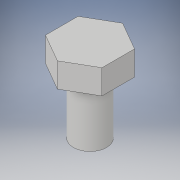
# Autodesk Inventor part: Crossbeam to LS Bolt
Saved by Autodesk Inventor 2017 (Build 210142000, 142)
## iProperties
Created: 2016-09-26
Part Number: Crossbeam to LS Bolt
Material: Generic
Document SubType Name: Modeling
Designer: Hanson
Density: 1 g/cm^3
Appearance: Default
Author: Hanson
Autodesk Inventor part; units mm, degrees
ref_plane "YZ Plane" through (0, 0, 0) normal (1, 0, 0) x (0, 1, 0)
ref_plane "XZ Plane" through (0, 0, 0) normal (0, 1, 0) x (-1, 0, 0)
ref_plane "XY Plane" through (0, 0, 0) normal (0, 0, 1) x (1, 0, 0)
sketch "Sketch1" plane through (0, 0, 0) normal (0, 1, 0) x (-1, 0, 0)
  circle A0 centre (0, 0) radius 2.5781
  dimension "d0" = 5.1562
  constraints: 1 centre point, 1 coincident
  measures "d0" diameter of A0
extrude "Extrusion1" add sketch "Sketch1" along normal blind 14.224
sketch "Sketch2" plane through (0, 14.224, 0) normal (0, 1, 0) x (1, 0, 0)
  line L0 (0, 5.08) -> (4.3994, 2.54)
  line L1 (4.3994, 2.54) -> (4.3994, -2.54)
  line L2 (4.3994, -2.54) -> (0, -5.08)
  line L3 (0, -5.08) -> (-4.3994, -2.54)
  line L4 (-4.3994, -2.54) -> (-4.3994, 2.54)
  line L5 (-4.3994, 2.54) -> (0, 5.08)
  point P0 (0, 0)
  point P1 (0, 0)
  dimension "d3" = 5.08
  constraints: 12 end point, 1 coincident, 13 other
  measures "d3" distance of point (0, 0) L0.start
extrude "Extrusion2" add sketch "Sketch2" along normal blind 3.81
sketch "Sketch3" plane through (0, 0, 0) normal (0, -1, 0) x (1, 0, 0)
  circle A0 centre (0, 0) radius 2.5781
  constraints: 1 centre point, 1 coincident
extrude "Extrusion3" cut sketch "Sketch3" against normal blind 5.08
body "Solid1"
